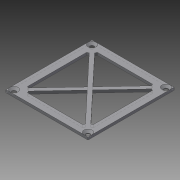
# Autodesk Inventor part: Mounting Plate
Saved by Autodesk Inventor 2015 (Build 190159000, 159)
## iProperties
Created: 2019-05-03
Part Number: Mounting Plate
Material: Generic
Document SubType Name: Modeling
Designer: Toby
Density: 1 g/cm^3
Appearance: Default
Author: Toby
Autodesk Inventor part; units mm, degrees
ref_plane "YZ Plane" through (0, 0, 0) normal (1, 0, 0) x (0, 1, 0)
ref_plane "XZ Plane" through (0, 0, 0) normal (0, 1, 0) x (-1, 0, 0)
ref_plane "XY Plane" through (0, 0, 0) normal (0, 0, 1) x (1, 0, 0)
sketch "Sketch1" plane through (0, 0, 0) normal (0, 0, 1) x (1, 0, 0)
  line L0 (-51.4052, 38.5707) -> (3.5948, 38.5707)
  line L1 (3.5948, 38.5707) -> (3.5948, -19.4293)
  line L2 (3.5948, -19.4293) -> (-51.4052, -19.4293)
  line L3 (-51.4052, -19.4293) -> (-51.4052, 38.5707)
  line L4 (-54.4052, 41.5707) -> (6.5948, 41.5707)
  line L5 (6.5948, 41.5707) -> (6.5948, -22.4293)
  line L6 (6.5948, -22.4293) -> (-54.4052, -22.4293)
  line L7 (-54.4052, -22.4293) -> (-54.4052, 41.5707)
  line L8 (-48.4052, 35.5707) -> (0.5948, 35.5707)
  line L9 (0.5948, 35.5707) -> (0.5948, -16.4293)
  line L10 (0.5948, -16.4293) -> (-48.4052, -16.4293)
  line L11 (-48.4052, -16.4293) -> (-48.4052, 35.5707)
  point P0 (0, 0)
  dimension "d0" = 55
  dimension "d1" = 58
  dimension "d2" = 3
  dimension "d3" = 3
  dimension "d4" = 3
  dimension "d5" = 3
  dimension "d6" = 3
  dimension "d7" = 3
  dimension "d8" = 3
  dimension "d9" = 3
  constraints: 24 end point, 6 parallel, 4 coincident, 3 horizontal, 3 perpendicular
  measures "d0" distance of L0.start L0.end
  measures "d1" distance of L2.end L0.start
  measures "d2" distance between parallel lines of L0 L4
  measures "d3" distance between parallel lines of L0 L8
  measures "d4" distance between parallel lines of L2 L10
  measures "d5" distance between parallel lines of L2 L6
  measures "d6" distance between parallel lines of L3 L7
  measures "d7" distance between parallel lines of L11 L3
  measures "d8" distance between parallel lines of L1 L9
  measures "d9" distance between parallel lines of L1 L5
extrude "Extrusion1" add sketch "Sketch1" along normal blind 2 contours L0 L1 L2 L3 | L4 L5 L6 L7
sketch "Sketch2" plane through (0, 0, 2) normal (0, 0, 1) x (1, 0, 0)
  line L0 (-54.4052, 41.5707) -> (-54.4052, -22.4293) projected
  line L1 (6.5948, 41.5707) -> (-54.4052, 41.5707) projected
  line L2 (6.5948, 41.5707) -> (6.5948, -22.4293) projected
  line L3 (-54.4052, -22.4293) -> (6.5948, -22.4293) projected
  point P0 (0, 0)
  point P1 (-51.4052, 38.5707)
  point P2 (3.5948, 38.5707)
  point P3 (3.5948, -19.4293)
  point P4 (-51.4052, -19.4293)
  dimension "d12" = 3
  dimension "d13" = 3
  dimension "d14" = 3
  dimension "d15" = 3
  dimension "d16" = 3
  dimension "d17" = 3
  dimension "d18" = 3
  dimension "d19" = 3
  measures "d12" distance from line of L0 point (-51.405, 38.571)
  measures "d13" distance from line of L1 point (-51.405, 38.571)
  measures "d14" distance from line of L1 point (3.595, 38.571)
  measures "d15" distance from line of L2 point (3.595, 38.571)
  measures "d16" distance from line of L2 point (3.595, -19.429)
  measures "d17" distance from line of L3 point (3.595, -19.429)
  measures "d18" distance from line of L3 point (-51.405, -19.429)
  measures "d19" distance from line of L0 point (-51.405, -19.429)
hole "Hole1" at (-51.4052, 38.5707, 2) at (3.5948, 38.5707, 2) at (3.5948, -19.4293, 2) at (-51.4052, -19.4293, 2) direction (0, 0, -1) diameter 3 depth 8 tip angle 118 countersink diameter 6 countersink angle 90
sketch "Sketch3" plane through (0, 0, 2) normal (0, 0, 1) x (1, 0, 0)
  line L0 (-48.4052, -16.4293) -> (-48.4052, 35.5707) projected
  line L1 (0.5948, 35.5707) -> (-48.4052, 35.5707) projected
  line L2 (0.5948, 35.5707) -> (0.5948, -16.4293) projected
  line L3 (-48.4052, -16.4293) -> (0.5948, -16.4293) projected
  line L4 (-48.4052, 33.5707) -> (-1.4052, -16.4293)
  line L5 (-1.4052, -16.4293) -> (0.5948, -16.4293)
  line L6 (0.5948, -16.4293) -> (0.5948, -14.4293)
  line L7 (0.5948, -14.4293) -> (-46.4052, 35.5707)
  line L8 (-48.4052, 35.5707) -> (-46.4052, 35.5707)
  line L9 (-48.4052, 35.5707) -> (-48.4052, 33.5707)
  line L10 (-48.4052, -14.4293) -> (-1.4052, 35.5707)
  line L11 (-1.4052, 35.5707) -> (0.5948, 35.5707)
  line L12 (0.5948, 33.5707) -> (-46.4052, -16.4293)
  line L13 (-46.4052, -16.4293) -> (-48.4052, -16.4293)
  line L14 (-48.4052, -16.4293) -> (-48.4052, -14.4293)
  point P0 (0, 0)
  point P1 (-46.4052, -16.4293)
  dimension "d27" = 2
  dimension "d28" = 2
  dimension "d29" = 2
  dimension "d30" = 2
  dimension "d31" = 2
  dimension "d32" = 2
  dimension "d33" = 2
  dimension "d34" = 2
  constraints: 22 end point, 9 point on line, 3 collinear, 2 parallel, 1 horizontal, 1 perpendicular
  measures "d27" distance from line of L1 L4.start
  measures "d28" horizontal distance of L4.start L7.end
  measures "d29" distance from line of L2 L10.end
  measures "d30" horizontal distance of L10.end L12.start
  measures "d31" distance from line of L0 point (-46.405, -16.429)
  measures "d32" distance from line of L3 L10.start
  measures "d33" horizontal distance of L4.end L6.end
  measures "d34" distance from line of L2 L4.end
extrude "Extrusion2" add sketch "Sketch3" against normal blind 2 contours L0 L10 L4 L12 L3 | L0 L1 L7 L10 L4 | L10 L7 L12 L4 | L4 L12 L7 L2 L3 | L10 L1 L2 L12 L7
chamfer "Chamfer1" distance 2 angle 45 8 edges at (-46.4052, 35.5707, 1) (-48.4052, 33.5707, 1) (0.5948, 33.5707, 1) (-1.4052, 35.5707, 1) (0.5948, -14.4293, 1) (-1.4052, -16.4293, 1) (-48.4052, -14.4293, 1) (-46.4052, -16.4293, 1)
body "Solid1"
